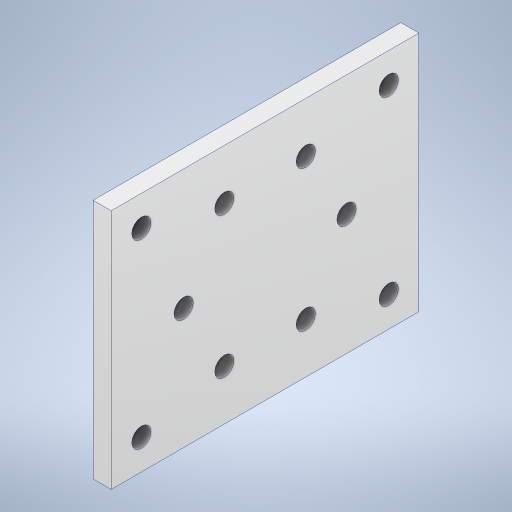
# Autodesk Inventor part: link5_plate2
Saved by Autodesk Inventor 2024 (Build 280153000, 153)
## iProperties
Created: 2024-12-13
Part Number: link5_plate2
Material: アルミニウム 6061
Document SubType Name: Modeling
Designer: hirek
Density: 2.7 g/cm^3
Appearance: アルミニウム - フラット
Mass: 37.9594 g
Surface Area: 106.915 cm^2
Volume: 14.059 cm^3
Author: hirek
Autodesk Inventor part; units mm, degrees
ref_plane "YZ Plane" through (0, 0, 0) normal (1, 0, 0) x (0, 1, 0)
ref_plane "XZ Plane" through (0, 0, 0) normal (0, 1, 0) x (-1, 0, 0)
ref_plane "XY Plane" through (0, 0, 0) normal (0, 0, 1) x (1, 0, 0)
sketch "スケッチ1" plane through (0, 0, 0) normal (1, 0, 0) x (0, 1, 0)
  line L0 (35, -49) -> (-5, -49)
  line L1 (-5, -49) -> (-5, -100)
  line L2 (-5, -100) -> (35, -100)
  line L3 (35, -100) -> (35, -49)
  dimension "d1" = 40
  dimension "d2" = 51
  constraints: 8 end point, 2 parallel, 1 horizontal, 1 perpendicular
  measures "d1" distance of L2.end L1.end
  measures "d2" distance of L1.end L0.end
extrude "押し出し1" add sketch "スケッチ1" along normal blind 3
sketch "スケッチ4" plane through (3, 0, 0) normal (1, 0, 0) x (0, 0, -1)
  line L0 (54, 30) -> (95, 30)
  line L1 (95, 30) -> (95, 0)
  line L2 (95, 0) -> (54, 0)
  line L3 (54, 0) -> (54, 30)
  line L4 (100, 35) -> (49, 35) projected
  line L5 (100, -5) -> (100, 35) projected
  point P0 (0, 0)
  dimension "d29" = 41
  dimension "d30" = 30
  dimension "d31" = 5
  dimension "d32" = 5
  constraints: 8 end point, 4 coincident, 2 parallel, 1 horizontal, 1 perpendicular
  measures "d29" distance of L1.end L2.end
  measures "d30" distance of L0.end L1.end
  measures "d31" distance between parallel lines of L0 L4
  measures "d32" distance between parallel lines of L5 L1
hole "穴2" at (3, 30, -54) at (3, 0, -54) at (3, 0, -95) at (3, 30, -95) direction (-1, 0, 0) diameter 3.2 end through all
sketch "スケッチ6" plane through (3, 0, 0) normal (1, 0, 0) x (0, 0, -1)
  line L0 (49, 35) -> (49, -5) projected
  line L1 (49, 15) -> (100, 15)
  line L2 (100, -5) -> (100, 35) projected
  circle A0 centre (74.5, 15) radius 13.5
  point P0 (0, 0)
  point P1 (88, 15)
  point P2 (81.25, 26.6913)
  point P3 (67.75, 26.6913)
  point P4 (61, 15)
  point P5 (67.75, 3.3087)
  point P6 (81.25, 3.3087)
  dimension "d53" = 27
  dimension "d56" = 360
  constraints: 3 midpoint, 2 end point, 1 horizontal alignment, 1 point on line, 9 other
hole "穴4" at (3, 15, -88) at (3, 26.6913, -81.25) at (3, 26.6913, -67.75) at (3, 15, -61) at (3, 3.3087, -67.75) at (3, 3.3087, -81.25) direction (-1, 0, 0) diameter 3.2 end through all
